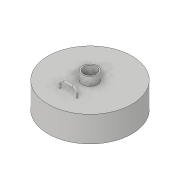
# Autodesk Inventor part: bulckhead
Saved by Autodesk Inventor 2019 (Build 230136000, 136)
## iProperties
Created: 2020-09-30
Part Number: bulckhead
Material: Generic
Document SubType Name: Modeling
Designer: Nikolas
Density: 1 g/cm^3
Appearance: Default
Author: Nikolas
Autodesk Inventor part; units mm, degrees
ref_plane "YZ Plane" through (0, 0, 0) normal (1, 0, 0) x (0, 1, 0)
ref_plane "XZ Plane" through (0, 0, 0) normal (0, 1, 0) x (-1, 0, 0)
ref_plane "XY Plane" through (0, 0, 0) normal (0, 0, 1) x (1, 0, 0)
sketch "Sketch1" plane through (0, 0, 0) normal (0, 0, 1) x (1, 0, 0)
  line L0 (1.5, 0) -> (1.5, 40)
  line L1 (3, 0) -> (3, 30)
  line L2 (3, 30) -> (9, 30)
  line L3 (9, 30) -> (9, 40)
  line L4 (9, 40) -> (10.5, 40)
  line L5 (10.5, 40) -> (10.5, 30)
  line L6 (10.5, 30) -> (50.5, 30)
  line L7 (50.5, 30) -> (50.5, 0)
  line L8 (50.5, 0) -> (3, 0)
  point P0 (0, 0)
  constraints: 18 end point, 6 perpendicular, 1 horizontal
revolve "Revolution1" add sketch "Sketch1" angle 360 about axis through (1.5, 0, 0) along (0, 1, 0)
sketch "Sketch2" plane through (1.5, 30, 0) normal (0, 1, 0) x (1, 0, 0)
  point P0 (-1.5, 0)
sketch "Sketch4" plane through (1.5, 30, 0) normal (0, 1, 0) x (1, 0, 0)
  circle A0 centre (0, 0) radius 1.5 projected
  circle A1 centre (-10, -25) radius 1
  point P0 (-1.5, 0)
  constraints: 1 centre point, 1 horizontal alignment
sketch3d "3D Sketch3"
  line L0 (-8.5, 30, 25) -> (-8.5, 34, 25)
  arc A0 (-8.5, 34, 25) -> (-3.5, 39, 25) centre (-3.5, 34, 25) ccw
  line L1 (-3.5, 39, 25) -> (6.5, 39, 25)
  arc A1 (6.5, 39, 25) -> (11.5, 34, 25) centre (6.5, 34, 25) ccw
  line L2 (11.5, 34, 25) -> (11.5, 30, 25)
  dimension "d21" = 5
  dimension "d22" = 5
sweep "Sweep2" add profiles "Sketch4" path "3D Sketch3" contours A1
equation "\"d22\" = d21"
body "Solid1"
